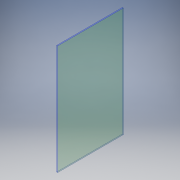
# Autodesk Inventor part: SideEBoard
Saved by Autodesk Inventor 2019 (Build 230136000, 136)
## iProperties
Created: 2020-01-24
Part Number: SideEBoard
Material: Generic
Document SubType Name: Modeling
Designer: james
Density: 1 g/cm^3
Appearance: Clear - Blue
Author: james
Autodesk Inventor part; units mm, degrees
ref_plane "YZ Plane" through (0, 0, 0) normal (1, 0, 0) x (0, 1, 0)
ref_plane "XZ Plane" through (0, 0, 0) normal (0, 1, 0) x (-1, 0, 0)
ref_plane "XY Plane" through (0, 0, 0) normal (0, 0, 1) x (1, 0, 0)
sketch "Sketch1" plane through (0, 0, 0) normal (1, 0, 0) x (0, 1, 0)
  line L0 (390.3881, 109.7885) -> (-117.6119, 109.7885)
  line L1 (-117.6119, 109.7885) -> (-117.6119, -195.0115)
  line L2 (-117.6119, -195.0115) -> (390.3881, -195.0115)
  line L3 (390.3881, -195.0115) -> (390.3881, 109.7885)
  point P0 (0, 0)
  dimension "d0" = 304.8
  dimension "d1" = 508
  constraints: 8 end point, 2 parallel, 1 horizontal, 1 perpendicular
  measures "d0" distance of L0.end L1.end
  measures "d1" distance of L0.start L0.end
extrude "Extrusion1" add sketch "Sketch1" along normal blind 4.7625
body "Solid1"
